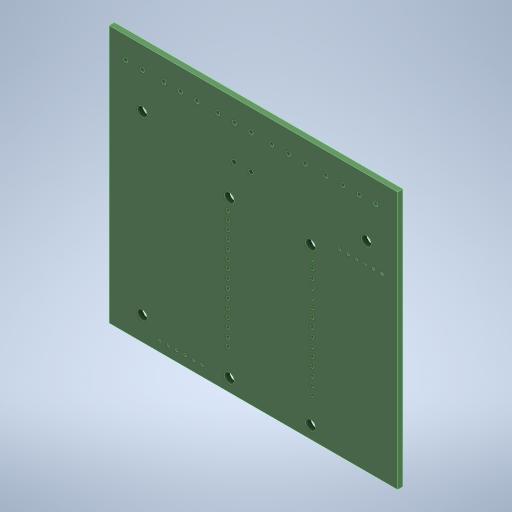
# Autodesk Inventor part: Modulo_DEC.kicad_pcb
Saved by Autodesk Inventor 2023 (Build 270158000, 158)
## iProperties
Created: 2023-12-31
Part Number: Modulo_DEC.kicad_pcb
Material: Generic
Document SubType Name: Modeling
Designer: Usuario
Density: 1 g/cm^3
Appearance: Board Outline
Author: Usuario
Autodesk Inventor part; units mm, degrees
ref_plane "YZ Plane" through (0, 0, 0) normal (1, 0, 0) x (0, 1, 0)
ref_plane "XZ Plane" through (0, 0, 0) normal (0, 1, 0) x (-1, 0, 0)
ref_plane "XY Plane" through (0, 0, 0) normal (0, 0, 1) x (1, 0, 0)
sketch "Sketch1" plane through (0, 0, 0) normal (0, 0, 1) x (1, 0, 0)
  line L0 (190.01, 101.6) -> (103.121, 101.6)
  line L1 (103.121, 101.6) -> (103.121, 24)
  line L2 (103.121, 24) -> (190.01, 24)
  line L3 (190.01, 24) -> (190.01, 101.6)
  circle A0 centre (180.571, 84.064) radius 1.5
  circle A1 centre (113.096, 84.014) radius 1.5
  circle A2 centre (113.096, 31.014) radius 1.5
  circle A3 centre (168.406, 95.094) radius 0.66
  circle A4 centre (173.406, 95.094) radius 0.66
  circle A5 centre (178.406, 95.094) radius 0.66
  circle A6 centre (183.406, 95.094) radius 0.66
  circle A7 centre (152.121, 95.089) radius 0.66
  circle A8 centre (157.121, 95.089) radius 0.66
  circle A9 centre (162.121, 95.089) radius 0.66
  circle A10 centre (135.871, 95.089) radius 0.66
  circle A11 centre (140.871, 95.089) radius 0.66
  circle A12 centre (145.871, 95.089) radius 0.66
  circle A13 centre (119.586, 95.094) radius 0.66
  circle A14 centre (124.586, 95.094) radius 0.66
  circle A15 centre (129.586, 95.094) radius 0.66
  circle A16 centre (108.096, 95.014) radius 0.66
  circle A17 centre (113.096, 95.014) radius 0.66
  circle A18 centre (140.746, 84.684) radius 0.7
  circle A19 centre (145.826, 84.684) radius 0.7
  circle A20 centre (118.436, 27.064) radius 0.4
  circle A21 centre (120.976, 27.064) radius 0.4
  circle A22 centre (123.516, 27.064) radius 0.4
  circle A23 centre (126.056, 27.064) radius 0.4
  circle A24 centre (128.596, 27.064) radius 0.4
  circle A25 centre (131.136, 27.064) radius 0.4
  circle A26 centre (185.311, 77.939) radius 0.4
  circle A27 centre (182.771, 77.939) radius 0.4
  circle A28 centre (180.231, 77.939) radius 0.4
  circle A29 centre (177.691, 77.939) radius 0.4
  circle A30 centre (175.151, 77.939) radius 0.4
  circle A31 centre (172.611, 77.939) radius 0.4
  circle A32 centre (164.23, 35.66) radius 0.51
  circle A33 centre (164.23, 38.2) radius 0.51
  circle A34 centre (164.23, 40.74) radius 0.51
  circle A35 centre (164.23, 43.28) radius 0.51
  circle A36 centre (164.23, 45.82) radius 0.51
  circle A37 centre (164.23, 48.36) radius 0.51
  circle A38 centre (164.23, 50.9) radius 0.51
  circle A39 centre (164.23, 53.44) radius 0.51
  circle A40 centre (164.23, 55.98) radius 0.51
  circle A41 centre (164.23, 58.52) radius 0.51
  circle A42 centre (164.23, 61.06) radius 0.51
  circle A43 centre (164.23, 63.6) radius 0.51
  circle A44 centre (164.23, 66.14) radius 0.51
  circle A45 centre (164.23, 68.68) radius 0.51
  circle A46 centre (164.23, 71.22) radius 0.51
  circle A47 centre (138.83, 71.22) radius 0.51
  circle A48 centre (138.83, 68.68) radius 0.51
  circle A49 centre (138.83, 66.14) radius 0.51
  circle A50 centre (138.83, 63.6) radius 0.51
  circle A51 centre (138.83, 61.06) radius 0.51
  circle A52 centre (138.83, 58.52) radius 0.51
  circle A53 centre (138.83, 55.98) radius 0.51
  circle A54 centre (138.83, 53.44) radius 0.51
  circle A55 centre (138.83, 50.9) radius 0.51
  circle A56 centre (138.83, 48.36) radius 0.51
  circle A57 centre (138.83, 45.82) radius 0.51
  circle A58 centre (138.83, 43.28) radius 0.51
  circle A59 centre (138.83, 40.74) radius 0.51
  circle A60 centre (138.83, 38.2) radius 0.51
  circle A61 centre (138.83, 35.66) radius 0.51
  circle A62 centre (163.81, 27.7) radius 1.5
  circle A63 centre (163.81, 74.65) radius 1.5
  circle A64 centre (139.3, 27.7) radius 1.5
  circle A65 centre (139.3, 74.65) radius 1.5
  line L4 (190.01, 27.7) -> (190.01, 24)
  point P0 (146.5655, 62.8)
  constraints: 66 centre point, 10 end point
extrude "Modulo_DEC.kicad_pcb_Outline" add sketch "Sketch1" along normal blind 1.6
body "Solid1"
